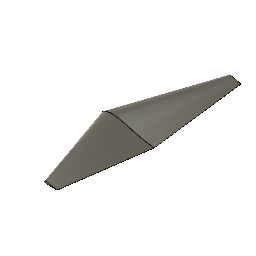
Aile_volante (Autodesk Fusion 360 design; units mm, degrees)
Autodesk Fusion 360 part; units mm, degrees
sketch "Esquisse2" plane through (0, 0, 0) normal (0, 1, 0) x (1, 0, 0)
  spline S0 degree 5 poles (199.2389, 17.4311) (199.2415, 17.3643) (199.1206, 17.225) (198.5619, 16.9995) (197.0938, 16.667) (194.2495, 16.2075) (190.6685, 15.7156) (186.6602, 15.2042) (182.5299, 14.6853) (178.5411, 14.1686) (174.8714, 13.6598) (171.585, 13.1588) (168.6633, 12.6619) (166.0277, 12.1628) (163.564, 11.6542) (161.1478, 11.129) (158.6667, 10.5816) (156.0493, 10.0096) (153.2739, 9.4141) (150.3532, 8.7983) (147.325, 8.1665) (144.2402, 7.5232) (141.1523, 6.8717) (138.1067, 6.2136) (135.1277, 5.5471) (132.2185, 4.8673) (129.3682, 4.1684) (126.5567, 3.4439) (123.7598, 2.6886) (120.9553, 1.8995) (118.1274, 1.0767) (115.2735, 0.2256) (112.4006, -0.645) (109.5221, -1.5241) (106.6529, -2.4) (103.8061, -3.2616) (100.989, -4.1001) (98.1989, -4.9101) (95.4194, -5.6915) (92.6262, -6.4475) (89.7926, -7.1835) (86.8951, -7.9049) (83.9195, -8.6164) (80.8658, -9.3198) (77.7549, -10.0127) (74.6316, -10.6874) (71.5537, -11.333) (68.5832, -11.9373) (65.7763, -12.4887) (63.1737, -12.9778) (60.7923, -13.3997) (58.6126, -13.7558) (56.5799, -14.0538) (54.6242, -14.305) (52.6757, -14.5212) (50.6809, -14.7123) (48.6232, -14.8828) (46.519, -15.0322) (44.4, -15.1562) (42.2985, -15.2482) (40.2331, -15.3005) (38.1907, -15.3057) (36.1377, -15.2578) (34.0385, -15.1528) (31.8705, -14.9893) (29.6406, -14.7702) (27.4018, -14.5026) (25.2306, -14.197) (23.2053, -13.8656) (21.384, -13.5214) (19.7809, -13.1763) (18.3496, -12.8402) (17.0115, -12.5116) (15.6797, -12.1732) (14.2863, -11.7792) (12.7968, -11.2738) (11.2167, -10.6247) (9.6011, -9.8533) (8.0608, -9.0631) (6.7038, -8.3594) (5.5912, -7.7928) (4.6643, -7.262) (3.762, -6.536) (2.7557, -5.432) (1.7001, -4.0099) (0.8029, -2.5462) (0.2492, -1.3296) (0.0696, -0.5092) (-0.0083, 0.0763) (-0.1167, 0.6989) (0.0954, 1.5811) (0.7989, 2.7024) (1.7815, 3.7896) (2.7609, 4.5609) (3.6495, 4.9748) (4.6093, 5.2532) (5.8063, 5.6217) (7.2431, 6.1216) (8.8187, 6.6791) (10.399, 7.1837) (11.8945, 7.5788) (13.2858, 7.8806) (14.6004, 8.1356) (15.9033, 8.3938) (17.2821, 8.6802) (18.8195, 9.003) (20.5702, 9.3579) (22.5298, 9.7347) (24.6445, 10.1195) (26.8379, 10.498) (29.0325, 10.8573) (31.172, 11.1882) (33.2456, 11.4886) (35.2747, 11.7608) (37.295, 12.0105) (39.3408, 12.2441) (41.4274, 12.4672) (43.5375, 12.6827) (45.6382, 12.892) (47.6967, 13.0959) (49.6947, 13.2957) (51.6461, 13.4941) (53.6037, 13.6957) (55.6379, 13.906) (57.8205, 14.1302) (60.2089, 14.3727) (62.8252, 14.6356) (65.6539, 14.9188) (68.6544, 15.2205) (71.7697, 15.5373) (74.9368, 15.8648) (78.0964, 16.1982) (81.2023, 16.5325) (84.2327, 16.8627) (87.1881, 17.1844) (90.0835, 17.4937) (92.9437, 17.787) (95.7964, 18.0616) (98.6668, 18.3153) (101.5714, 18.5467) (104.5117, 18.7553) (107.4788, 18.9412) (110.4572, 19.1051) (113.4296, 19.2482) (116.3807, 19.372) (119.3016, 19.4782) (122.1944, 19.5685) (125.0752, 19.6444) (127.9669, 19.7075) (130.8944, 19.7589) (133.8788, 19.7992) (136.9314, 19.8286) (140.0488, 19.8468) (143.2058, 19.8523) (146.356, 19.8434) (149.4457, 19.8179) (152.4236, 19.7738) (155.2528, 19.7099) (157.9218, 19.626) (160.4544, 19.5235) (162.9254, 19.4057) (165.4485, 19.2776) (168.1485, 19.1446) (171.1387, 19.0118) (174.4961, 18.8827) (178.2365, 18.7585) (182.2922, 18.6369) (186.4818, 18.5112) (190.5405, 18.3713) (194.1629, 18.2056) (197.0408, 18.0022) (198.5313, 17.8014) (199.1055, 17.6261) (199.2364, 17.498) (199.2389, 17.4311) knots 0 0 0 0 0 0 0.00588235 0.01176471 0.01764706 0.02352941 0.02941176 0.03529412 0.04117647 0.04705882 0.05294118 0.05882353 0.06470588 0.07058824 0.07647059 0.08235294 0.08823529 0.09411765 0.1 0.10588235 0.11176471 0.11764706 0.12352941 0.12941176 0.13529412 0.14117647 0.14705882 0.15294118 0.15882353 0.16470588 0.17058824 0.17647059 0.18235294 0.18823529 0.19411765 0.2 0.20588235 0.21176471 0.21764706 0.22352941 0.22941176 0.23529412 0.24117647 0.24705882 0.25294118 0.25882353 0.26470588 0.27058824 0.27647059 0.28235294 0.28823529 0.29411765 0.3 0.30588235 0.31176471 0.31764706 0.32352941 0.32941176 0.33529412 0.34117647 0.34705882 0.35294118 0.35882353 0.36470588 0.37058824 0.37647059 0.38235294 0.38823529 0.39411765 0.4 0.40588235 0.41176471 0.41764706 0.42352941 0.42941176 0.43529412 0.44117647 0.44705882 0.45294118 0.45882353 0.46470588 0.47058824 0.47647059 0.48235294 0.48823529 0.49411765 0.5 0.50588235 0.51176471 0.51764706 0.52352941 0.52941176 0.53529412 0.54117647 0.54705882 0.55294118 0.55882353 0.56470588 0.57058824 0.57647059 0.58235294 0.58823529 0.59411765 0.6 0.60588235 0.61176471 0.61764706 0.62352941 0.62941176 0.63529412 0.64117647 0.64705882 0.65294118 0.65882353 0.66470588 0.67058824 0.67647059 0.68235294 0.68823529 0.69411765 0.7 0.70588235 0.71176471 0.71764706 0.72352941 0.72941176 0.73529412 0.74117647 0.74705882 0.75294118 0.75882353 0.76470588 0.77058824 0.77647059 0.78235294 0.78823529 0.79411765 0.8 0.80588235 0.81176471 0.81764706 0.82352941 0.82941176 0.83529412 0.84117647 0.84705882 0.85294118 0.85882353 0.86470588 0.87058824 0.87647059 0.88235294 0.88823529 0.89411765 0.9 0.90588235 0.91176471 0.91764706 0.92352941 0.92941176 0.93529412 0.94117647 0.94705882 0.95294118 0.95882353 0.96470588 0.97058824 0.97647059 0.98235294 0.98823529 0.99411765 1 1 1 1 1 1
  point P0 (179.4787, 14.285)
  point P1 (159.7509, 10.8208)
  point P2 (140.0964, 6.6412)
  point P3 (120.513, 1.7659)
  point P4 (101.0293, -4.0831)
  point P5 (81.4682, -9.177)
  point P6 (61.7995, -13.2175)
  point P7 (51.899, -14.5918)
  point P8 (41.9253, -15.2507)
  point P9 (31.8561, -14.9755)
  point P10 (21.671, -13.5675)
  point P11 (16.5296, -12.3865)
  point P12 (11.3313, -10.6491)
  point P13 (6.0416, -8.0172)
  point P14 (3.3275, -6.0256)
  point P15 (0.3492, -1.4503)
  point P16 (0.0707, 1.2724)
  point P17 (2.2865, 4.1499)
  point P18 (4.6813, 5.2786)
  point P19 (9.536, 6.8998)
  point P20 (14.4334, 8.1037)
  point P21 (19.3511, 9.1089)
  point P22 (29.2109, 10.8807)
  point P23 (39.1154, 12.2153)
  point P24 (49.0525, 13.2319)
  point P25 (58.9896, 14.2485)
  point P26 (78.8637, 16.2818)
  point P27 (98.7378, 18.315)
  point P28 (118.7034, 19.4539)
  point P29 (138.7463, 19.8376)
  point P30 (158.8543, 19.5853)
  point P31 (179.0232, 18.7368)
ref_plane "Plan de construction1" through (99.5942, 350, -2.2753) normal (0, 1, 0) x (1, 0, 0)
sketch "Esquisse4" plane through (99.5942, 350, -2.2753) normal (0, 1, 0) x (1, 0, 0)
  spline S0 degree 5 poles (80.8739, -11.6794) (80.8746, -11.6962) (80.844, -11.7312) (80.7028, -11.788) (80.3319, -11.8716) (79.6139, -11.9873) (78.7109, -12.111) (77.7016, -12.2397) (76.6634, -12.3701) (75.663, -12.4999) (74.7443, -12.6277) (73.9227, -12.7536) (73.1927, -12.8784) (72.5336, -13.004) (71.916, -13.132) (71.3085, -13.2644) (70.6828, -13.4024) (70.0219, -13.5466) (69.321, -13.6968) (68.584, -13.852) (67.8209, -14.0111) (67.0448, -14.1731) (66.2693, -14.337) (65.5055, -14.5026) (64.7588, -14.6704) (64.0296, -14.8418) (63.3147, -15.0182) (62.6089, -15.2013) (61.9059, -15.3923) (61.2002, -15.5919) (60.4883, -15.7999) (59.7699, -16.0147) (59.0472, -16.2341) (58.3237, -16.4552) (57.6033, -16.6749) (56.889, -16.8906) (56.1824, -17.1001) (55.4822, -17.3024) (54.7835, -17.4974) (54.0801, -17.6863) (53.3651, -17.8705) (52.6328, -18.0512) (51.8803, -18.2296) (51.1085, -18.406) (50.3242, -18.5794) (49.5399, -18.7476) (48.7709, -18.9078) (48.0328, -19.0567) (47.3395, -19.1916) (46.7, -19.3103) (46.1166, -19.4118) (45.5819, -19.497) (45.0805, -19.5682) (44.5939, -19.6284) (44.1051, -19.6805) (43.6023, -19.7268) (43.084, -19.768) (42.5556, -19.8039) (42.0258, -19.8331) (41.5022, -19.8538) (40.9877, -19.864) (40.4771, -19.862) (39.9614, -19.8463) (39.4319, -19.8161) (38.8844, -19.7713) (38.3237, -19.7128) (37.7655, -19.6429) (37.23, -19.5644) (36.7362, -19.4804) (36.2968, -19.3942) (35.9112, -19.3088) (35.5647, -19.2261) (35.2362, -19.1449) (34.9042, -19.0593) (34.5535, -18.9564) (34.1776, -18.8231) (33.7805, -18.6533) (33.3795, -18.4574) (33.0039, -18.2633) (32.6788, -18.0953) (32.4157, -17.9615) (32.1927, -17.8277) (31.9687, -17.6362) (31.7161, -17.3478) (31.4564, -16.9884) (31.242, -16.6288) (31.1168, -16.3393) (31.08, -16.1496) (31.0621, -16.016) (31.035, -15.8719) (31.0806, -15.6631) (31.2454, -15.3903) (31.4828, -15.1177) (31.7246, -14.916) (31.9419, -14.8053) (32.17, -14.7369) (32.4531, -14.6526) (32.7995, -14.5338) (33.1866, -14.396) (33.5817, -14.2658) (33.9585, -14.1618) (34.309, -14.0826) (34.6374, -14.0181) (34.958, -13.9554) (35.2921, -13.8866) (35.6618, -13.8088) (36.0833, -13.7223) (36.56, -13.6294) (37.0805, -13.5333) (37.6265, -13.4377) (38.1778, -13.3461) (38.7178, -13.2612) (39.2406, -13.184) (39.7502, -13.1142) (40.2551, -13.0505) (40.7645, -12.9912) (41.284, -12.9348) (41.8112, -12.8804) (42.3384, -12.8277) (42.8567, -12.7763) (43.3601, -12.7261) (43.8497, -12.6766) (44.3368, -12.6265) (44.8386, -12.5746) (45.3739, -12.5195) (45.9586, -12.46) (46.6011, -12.3953) (47.2994, -12.3254) (48.0445, -12.2506) (48.8225, -12.1718) (49.6174, -12.0899) (50.4136, -12.0062) (51.1984, -11.9221) (51.9645, -11.8388) (52.7112, -11.7574) (53.4415, -11.6789) (54.1614, -11.6044) (54.8781, -11.5344) (55.5981, -11.4696) (56.3263, -11.4105) (57.0638, -11.357) (57.8086, -11.3094) (58.5571, -11.2673) (59.3048, -11.2305) (60.0477, -11.1986) (60.7831, -11.1713) (61.5111, -11.148) (62.2353, -11.1285) (62.9614, -11.1122) (63.6957, -11.0989) (64.4438, -11.0885) (65.209, -11.0808) (65.991, -11.0759) (66.7839, -11.0741) (67.5766, -11.076) (68.3552, -11.082) (69.1067, -11.0926) (69.8213, -11.1083) (70.4952, -11.1289) (71.1338, -11.1544) (71.7551, -11.1838) (72.3875, -11.2159) (73.0627, -11.2492) (73.8099, -11.2827) (74.6493, -11.3152) (75.5858, -11.3464) (76.6031, -11.377) (77.6562, -11.4085) (78.6783, -11.4436) (79.5918, -11.4851) (80.3184, -11.536) (80.695, -11.5864) (80.8402, -11.6304) (80.8733, -11.6626) (80.8739, -11.6794) knots 0 0 0 0 0 0 0.00588235 0.01176471 0.01764706 0.02352941 0.02941176 0.03529412 0.04117647 0.04705882 0.05294118 0.05882353 0.06470588 0.07058824 0.07647059 0.08235294 0.08823529 0.09411765 0.1 0.10588235 0.11176471 0.11764706 0.12352941 0.12941176 0.13529412 0.14117647 0.14705882 0.15294118 0.15882353 0.16470588 0.17058824 0.17647059 0.18235294 0.18823529 0.19411765 0.2 0.20588235 0.21176471 0.21764706 0.22352941 0.22941176 0.23529412 0.24117647 0.24705882 0.25294118 0.25882353 0.26470588 0.27058824 0.27647059 0.28235294 0.28823529 0.29411765 0.3 0.30588235 0.31176471 0.31764706 0.32352941 0.32941176 0.33529412 0.34117647 0.34705882 0.35294118 0.35882353 0.36470588 0.37058824 0.37647059 0.38235294 0.38823529 0.39411765 0.4 0.40588235 0.41176471 0.41764706 0.42352941 0.42941176 0.43529412 0.44117647 0.44705882 0.45294118 0.45882353 0.46470588 0.47058824 0.47647059 0.48235294 0.48823529 0.49411765 0.5 0.50588235 0.51176471 0.51764706 0.52352941 0.52941176 0.53529412 0.54117647 0.54705882 0.55294118 0.55882353 0.56470588 0.57058824 0.57647059 0.58235294 0.58823529 0.59411765 0.6 0.60588235 0.61176471 0.61764706 0.62352941 0.62941176 0.63529412 0.64117647 0.64705882 0.65294118 0.65882353 0.66470588 0.67058824 0.67647059 0.68235294 0.68823529 0.69411765 0.7 0.70588235 0.71176471 0.71764706 0.72352941 0.72941176 0.73529412 0.74117647 0.74705882 0.75294118 0.75882353 0.76470588 0.77058824 0.77647059 0.78235294 0.78823529 0.79411765 0.8 0.80588235 0.81176471 0.81764706 0.82352941 0.82941176 0.83529412 0.84117647 0.84705882 0.85294118 0.85882353 0.86470588 0.87058824 0.87647059 0.88235294 0.88823529 0.89411765 0.9 0.90588235 0.91176471 0.91764706 0.92352941 0.92941176 0.93529412 0.94117647 0.94705882 0.95294118 0.95882353 0.96470588 0.97058824 0.97647059 0.98235294 0.98823529 0.99411765 1 1 1 1 1 1
  point P0 (75.9338, -12.466)
  point P1 (71.0019, -13.332)
  point P2 (66.0883, -14.3769)
  point P3 (61.1924, -15.5957)
  point P4 (56.3215, -17.058)
  point P5 (51.4312, -18.3315)
  point P6 (46.514, -19.3416)
  point P7 (44.0389, -19.6852)
  point P8 (41.5455, -19.8499)
  point P9 (39.0282, -19.7811)
  point P10 (36.4819, -19.4291)
  point P11 (35.1966, -19.1338)
  point P12 (33.897, -18.6995)
  point P13 (32.5746, -18.0415)
  point P14 (31.8961, -17.5436)
  point P15 (31.1515, -16.3998)
  point P16 (31.0642, -16.0372)
  point P17 (31.0818, -15.7191)
  point P18 (31.6358, -14.9997)
  point P19 (32.2345, -14.7176)
  point P20 (33.4482, -14.3123)
  point P21 (34.6725, -14.0113)
  point P22 (35.902, -13.76)
  point P23 (38.3669, -13.317)
  point P24 (40.843, -12.9834)
  point P25 (43.3273, -12.7292)
  point P26 (45.8116, -12.4751)
  point P27 (50.7801, -11.9668)
  point P28 (55.7486, -11.4585)
  point P29 (60.74, -11.1737)
  point P30 (65.7508, -11.0778)
  point P31 (70.7777, -11.1409)
  point P32 (75.82, -11.353)
loft "Lissage1" add profiles "Esquisse2", "Esquisse4" section 1 section 2 makes body 1
mirror "Symétrie miroir1" about plane through (0, 0, 0) normal (0, 1, 0) of bodies 1 makes body 2
copy_body "Corps->Comp1" bodies 1 removing the originals makes body 3 in component "aile_droite"
copy_body "Corps->Comp2" bodies 2 removing the originals makes body 4 in component "aile_gauche"
component "aile_droite" placed x (1, 0, 0) y (0, 1, 0) z (0, 0, 1) at (0, 0, 0)
component "aile_gauche" placed x (1, 0, 0) y (0, 1, 0) z (0, 0, 1) at (0, 0, 0)
named bodies: "aile_droite", "aile_gauche"
